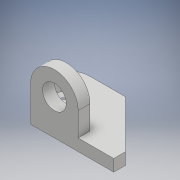
# Autodesk Inventor part: 25
Saved by Autodesk Inventor 2017 (Build 210142000, 142)
## iProperties
Part Number: 25
Material: 一般
Document SubType Name: Modeling
Designer: Brian
Density: 1 g/cm^3
Appearance: 預設
Author: Brian
Autodesk Inventor part; units mm, degrees
ref_plane "YZ Plane" through (0, 0, 0) normal (1, 0, 0) x (0, 1, 0)
ref_plane "XZ Plane" through (0, 0, 0) normal (0, 1, 0) x (-1, 0, 0)
ref_plane "XY Plane" through (0, 0, 0) normal (0, 0, 1) x (1, 0, 0)
sketch "草圖1" plane through (0, 0, 0) normal (0, 1, 0) x (-1, 0, 0)
  line L0 (0, 0) -> (-40, 0)
  line L1 (-40, 0) -> (-40, -40)
  line L2 (-40, -40) -> (0, -40)
  line L3 (0, -40) -> (0, 0)
  dimension "d0" = 40
  dimension "d1" = 40
  constraints: 8 end point, 2 parallel, 1 horizontal, 1 perpendicular
  measures "d0" distance of L1.end L2.end
  measures "d1" distance of L2.end L0.start
extrude "擠出1" add sketch "草圖1" along normal blind 10
sketch "草圖2" plane through (40, 0, -40) normal (0, 0, -1) x (-1, 0, 0)
  line L0 (40, 0) -> (0, 0) projected
  line L1 (40, 0) -> (-30, 0)
  line L2 (-30, 0) -> (-30, 50)
  line L3 (-30, 50) -> (40, 50)
  line L4 (40, 50) -> (40, 0)
  line L5 (40, 10) -> (0, 10) projected
  line L6 (40, 10) -> (60, 10)
  line L7 (60, 10) -> (60, 50)
  line L8 (60, 50) -> (40, 50)
  line L9 (40, 50) -> (40, 10)
  line L10 (0, 0) -> (0, 10) projected
  dimension "d4" = 40
  dimension "d5" = 30
  dimension "d6" = 20
  constraints: 16 end point, 4 parallel, 2 horizontal, 2 perpendicular, 1 point on line
  measures "d4" distance of L6.end L7.end
  measures "d5" distance between parallel lines of L2 L10
  measures "d6" distance of L5.start L6.end
extrude "擠出2" add sketch "草圖2" along normal blind 10
fillet "圓角1" radius 20 2 edges at (-20, 50, -45) (-20, 10, -45)
chamfer "倒角1" distance 40 angle 45 1 edges at (70, 50, -45)
fillet "圓角2" radius 20 2 edges at (0, 5, 0) (40, 5, 0)
hole "孔1" at (20, 10, -20) direction (0, -1, 0) diameter 20 depth 10 tip angle 118
hole "孔2" at (0, 30, -40) direction (0, 0, -1) diameter 20 depth 8 tip angle 118
